Autodesk Fusion 360 part; units mm, degrees
(part 5 of 5)
  spline S1555 degree 3 poles (12.9782, 1.8894) (13.0053, 1.745) (13.1136, 1.5194) (13.2129, 1.4021) knots 0 0 0 0 1 1 1 1
  spline S1556 degree 3 poles (13.2129, 1.4021) (13.3122, 1.2667) (13.3844, 1.0411) (13.3844, 0.8335) knots 0 0 0 0 1 1 1 1
  spline S1557 degree 3 poles (13.3844, 0.8335) (13.3844, 0.6349) (13.4205, 0.4815) (13.4746, 0.4815) knots 0 0 0 0 1 1 1 1
  spline S1558 degree 3 poles (13.4746, 0.4815) (13.5288, 0.4815) (13.5649, 0.8245) (13.5649, 1.3389) knots 0 0 0 0 1 1 1 1
  spline S1559 degree 3 poles (13.2039, 0.7523) (13.2039, 0.8696) (13.1587, 0.9147) (13.0685, 0.8786) knots 0 0 0 0 1 1 1 1
  spline S1560 degree 3 poles (13.0685, 0.8786) (12.9602, 0.8335) (12.9512, 0.7884) (13.0324, 0.6981) knots 0 0 0 0 1 1 1 1
  spline S1561 degree 3 poles (13.0324, 0.6981) (13.1678, 0.5266) (13.2039, 0.5357) (13.2039, 0.7523) knots 0 0 0 0 1 1 1 1
  spline S1562 degree 3 poles (10.5866, 1.2577) (10.5234, 1.4021) (10.5234, 1.5465) (10.5866, 1.6548) knots 0 0 0 0 1 1 1 1
  spline S1563 degree 3 poles (10.5866, 1.6548) (10.7039, 1.8714) (10.7039, 2.1963) (10.5956, 2.1963) knots 0 0 0 0 1 1 1 1
  spline S1564 degree 3 poles (10.5956, 2.1963) (10.5505, 2.1963) (10.4783, 2.2775) (10.4512, 2.3858) knots 0 0 0 0 1 1 1 1
  spline S1565 degree 3 poles (10.4512, 2.3858) (10.3971, 2.5573) (10.3881, 2.5663) (10.2707, 2.4038) knots 0 0 0 0 1 1 1 1
  spline S1566 degree 3 poles (10.2707, 2.4038) (10.1895, 2.3046) (10.1805, 2.2053) (10.2346, 2.1602) knots 0 0 0 0 1 1 1 1
  spline S1567 degree 3 poles (10.2346, 2.1602) (10.2798, 2.106) (10.3159, 1.9345) (10.3159, 1.7721) knots 0 0 0 0 1 1 1 1
  spline S1568 degree 3 poles (10.3159, 1.7721) (10.3159, 1.4562) (10.4783, 1.023) (10.5956, 1.023) knots 0 0 0 0 1 1 1 1
  spline S1569 degree 3 poles (10.5956, 1.023) (10.6408, 1.023) (10.6317, 1.1313) (10.5866, 1.2577) knots 0 0 0 0 1 1 1 1
  spline S1570 degree 3 poles (12.8338, 1.5284) (12.8338, 1.6277) (12.8068, 1.6548) (12.7797, 1.5826) knots 0 0 0 0 1 1 1 1
  spline S1571 degree 3 poles (12.7797, 1.5826) (12.7526, 1.5194) (12.7616, 1.4382) (12.7887, 1.4111) knots 0 0 0 0 1 1 1 1
  spline S1572 degree 3 poles (12.7887, 1.4111) (12.8158, 1.375) (12.8429, 1.4291) (12.8338, 1.5284) knots 0 0 0 0 1 1 1 1
  spline S1573 degree 3 poles (11.3537, 2.9002) (11.3176, 3.0356) (11.3718, 3.0897) (11.5974, 3.1619) knots 0 0 0 0 1 1 1 1
  line L88 (11.5974, 3.1619) -> (11.8952, 3.2612)
  line L89 (11.8952, 3.2612) -> (11.5794, 3.2702)
  spline S1574 degree 3 poles (11.5794, 3.2702) (11.2003, 3.2793) (10.5595, 3.0717) (10.5144, 2.9183) knots 0 0 0 0 1 1 1 1
  spline S1575 degree 3 poles (10.5144, 2.9183) (10.4873, 2.837) (10.5686, 2.819) (10.8032, 2.8461) knots 0 0 0 0 1 1 1 1
  spline S1576 degree 3 poles (10.8032, 2.8461) (10.9837, 2.8641) (11.1281, 2.8461) (11.1281, 2.81) knots 0 0 0 0 1 1 1 1
  spline S1577 degree 3 poles (11.1281, 2.81) (11.1281, 2.7739) (11.1913, 2.7378) (11.2725, 2.7378) knots 0 0 0 0 1 1 1 1
  spline S1578 degree 3 poles (11.2725, 2.7378) (11.3628, 2.7378) (11.3898, 2.7919) (11.3537, 2.9002) knots 0 0 0 0 1 1 1 1
  spline S1579 degree 3 poles (10.1083, 3.0175) (10.1263, 3.198) (10.1173, 3.198) (9.9458, 3.0536) knots 0 0 0 0 1 1 1 1
  spline S1580 degree 3 poles (9.9458, 3.0536) (9.7292, 2.8551) (9.7292, 2.828) (9.9368, 2.828) knots 0 0 0 0 1 1 1 1
  spline S1581 degree 3 poles (9.9368, 2.828) (10.0361, 2.828) (10.0993, 2.9002) (10.1083, 3.0175) knots 0 0 0 0 1 1 1 1
  spline S1582 degree 3 poles (13.2941, 3.0446) (13.2941, 3.198) (13.0865, 3.2883) (12.9331, 3.189) knots 0 0 0 0 1 1 1 1
  spline S1583 degree 3 poles (12.9331, 3.189) (12.8429, 3.1349) (12.8609, 3.0897) (13.0053, 3.0175) knots 0 0 0 0 1 1 1 1
  spline S1584 degree 3 poles (13.0053, 3.0175) (13.249, 2.8912) (13.2941, 2.8912) (13.2941, 3.0446) knots 0 0 0 0 1 1 1 1
  spline S1585 degree 3 poles (-8.6727, -4.41) (-8.6366, -4.3017) (-8.5825, -4.2115) (-8.5374, -4.2115) knots 0 0 0 0 1 1 1 1
  spline S1586 degree 3 poles (-8.5374, -4.2115) (-8.4922, -4.2115) (-8.4561, -4.1483) (-8.4561, -4.0671) knots 0 0 0 0 1 1 1 1
  spline S1587 degree 3 poles (-8.4561, -4.0671) (-8.4561, -3.9498) (-8.5103, -3.9678) (-8.6998, -4.1573) knots 0 0 0 0 1 1 1 1
  spline S1588 degree 3 poles (-8.6998, -4.1573) (-8.8803, -4.3469) (-8.9164, -4.4191) (-8.8262, -4.5093) knots 0 0 0 0 1 1 1 1
  spline S1589 degree 3 poles (-8.8262, -4.5093) (-8.7449, -4.5905) (-8.7088, -4.5725) (-8.6727, -4.41) knots 0 0 0 0 1 1 1 1
  spline S1590 degree 3 poles (-9.864, -4.41) (-9.837, -4.3559) (-9.855, -4.2837) (-9.9092, -4.2566) knots 0 0 0 0 1 1 1 1
  spline S1591 degree 3 poles (-9.9092, -4.2566) (-10.0445, -4.1664) (-10.1348, -4.2837) (-10.0175, -4.401) knots 0 0 0 0 1 1 1 1
  spline S1592 degree 3 poles (-10.0175, -4.401) (-9.9543, -4.4642) (-9.9001, -4.4642) (-9.864, -4.41) knots 0 0 0 0 1 1 1 1
  spline S1593 degree 3 poles (-8.6637, -3.4895) (-8.6818, -3.3) (-8.7449, -3.2548) (-9.142, -3.1646) knots 0 0 0 0 1 1 1 1
  spline S1594 degree 3 poles (-9.142, -3.1646) (-9.6023, -3.0653) (-9.6113, -3.0653) (-9.6113, -3.2729) knots 0 0 0 0 1 1 1 1
  spline S1595 degree 3 poles (-9.6113, -3.2729) (-9.6113, -3.4263) (-9.5572, -3.4895) (-9.4399, -3.4895) knots 0 0 0 0 1 1 1 1
  spline S1596 degree 3 poles (-9.4399, -3.4895) (-9.3496, -3.4895) (-9.2594, -3.5256) (-9.2233, -3.5797) knots 0 0 0 0 1 1 1 1
  spline S1597 degree 3 poles (-9.2233, -3.5797) (-9.1962, -3.6339) (-9.0879, -3.6339) (-8.9525, -3.5797) knots 0 0 0 0 1 1 1 1
  spline S1598 degree 3 poles (-8.9525, -3.5797) (-8.8081, -3.5256) (-8.7269, -3.5346) (-8.6908, -3.6068) knots 0 0 0 0 1 1 1 1
  spline S1599 degree 3 poles (-8.6908, -3.6068) (-8.6637, -3.67) (-8.6547, -3.6158) (-8.6637, -3.4895) knots 0 0 0 0 1 1 1 1
  spline S1600 degree 3 poles (24.9363, -2.6321) (24.9363, -2.5058) (24.9724, -2.4065) (25.0266, -2.4065) knots 0 0 0 0 1 1 1 1
  spline S1601 degree 3 poles (25.0266, -2.4065) (25.0717, -2.4065) (25.1168, -2.3704) (25.1168, -2.3162) knots 0 0 0 0 1 1 1 1
  spline S1602 degree 3 poles (25.1168, -2.3162) (25.1168, -2.1809) (24.9724, -2.2079) (24.81, -2.3704) knots 0 0 0 0 1 1 1 1
  spline S1603 degree 3 poles (24.81, -2.3704) (24.6295, -2.5509) (24.6205, -2.8577) (24.801, -2.8577) knots 0 0 0 0 1 1 1 1
  spline S1604 degree 3 poles (24.801, -2.8577) (24.8822, -2.8577) (24.9363, -2.7765) (24.9363, -2.6321) knots 0 0 0 0 1 1 1 1
  spline S1605 degree 3 poles (-26.3798, -2.587) (-26.1542, -2.5509) (-26.1812, -2.5238) (-26.6415, -2.4245) knots 0 0 0 0 1 1 1 1
  spline S1606 degree 3 poles (-26.6415, -2.4245) (-27.165, -2.2982) (-27.4086, -2.3614) (-27.2733, -2.578) knots 0 0 0 0 1 1 1 1
  spline S1607 degree 3 poles (-27.2733, -2.578) (-27.2191, -2.6772) (-26.8852, -2.6863) (-26.3798, -2.587) knots 0 0 0 0 1 1 1 1
  spline S1608 degree 3 poles (-24.1596, -2.4877) (-24.1596, -2.4155) (-24.4936, -2.3162) (-24.7282, -2.3162) knots 0 0 0 0 1 1 1 1
  spline S1609 degree 3 poles (-24.7282, -2.3162) (-24.8726, -2.3162) (-24.8726, -2.3343) (-24.7643, -2.4426) knots 0 0 0 0 1 1 1 1
  spline S1610 degree 3 poles (-24.7643, -2.4426) (-24.647, -2.5689) (-24.1596, -2.596) (-24.1596, -2.4877) knots 0 0 0 0 1 1 1 1
  spline S1611 degree 3 poles (-23.7084, -2.4065) (-23.7084, -2.3614) (-23.7535, -2.3162) (-23.7986, -2.3162) knots 0 0 0 0 1 1 1 1
  spline S1612 degree 3 poles (-23.7986, -2.3162) (-23.8528, -2.3162) (-23.8889, -2.3614) (-23.8889, -2.4065) knots 0 0 0 0 1 1 1 1
  spline S1613 degree 3 poles (-23.8889, -2.4065) (-23.8889, -2.4606) (-23.8528, -2.4967) (-23.7986, -2.4967) knots 0 0 0 0 1 1 1 1
  spline S1614 degree 3 poles (-23.7986, -2.4967) (-23.7535, -2.4967) (-23.7084, -2.4606) (-23.7084, -2.4065) knots 0 0 0 0 1 1 1 1
  spline S1615 degree 3 poles (-25.6758, -1.2242) (-25.5224, -1.0618) (-25.5224, -1.0527) (-25.6849, -1.0527) knots 0 0 0 0 1 1 1 1
  spline S1616 degree 3 poles (-25.6849, -1.0527) (-25.8924, -1.0527) (-26.5152, -1.3145) (-26.3256, -1.3235) knots 0 0 0 0 1 1 1 1
  spline S1617 degree 3 poles (-26.3256, -1.3235) (-26.2534, -1.3235) (-26.109, -1.3415) (-26.0098, -1.3686) knots 0 0 0 0 1 1 1 1
  spline S1618 degree 3 poles (-26.0098, -1.3686) (-25.9015, -1.3867) (-25.7661, -1.3325) (-25.6758, -1.2242) knots 0 0 0 0 1 1 1 1
  spline S1619 degree 3 poles (-26.3617, -0.8) (-26.3888, -0.7549) (-26.5693, -0.6917) (-26.7679, -0.6556) knots 0 0 0 0 1 1 1 1
  spline S1620 degree 3 poles (-26.7679, -0.6556) (-26.9664, -0.6286) (-27.1379, -0.5564) (-27.1559, -0.5022) knots 0 0 0 0 1 1 1 1
  spline S1621 degree 3 poles (-27.1559, -0.5022) (-27.2011, -0.3578) (-27.5079, -0.5203) (-27.4808, -0.6827) knots 0 0 0 0 1 1 1 1
  spline S1622 degree 3 poles (-27.4808, -0.6827) (-27.4628, -0.791) (-27.3184, -0.8361) (-26.8852, -0.8542) knots 0 0 0 0 1 1 1 1
  spline S1623 degree 3 poles (-26.8852, -0.8542) (-26.5513, -0.8722) (-26.3347, -0.8452) (-26.3617, -0.8) knots 0 0 0 0 1 1 1 1
  spline S1624 degree 3 poles (-23.9791, -0.6827) (-23.9791, -0.6376) (-24.0243, -0.6195) (-24.0694, -0.6466) knots 0 0 0 0 1 1 1 1
  spline S1625 degree 3 poles (-24.0694, -0.6466) (-24.1235, -0.6737) (-24.1596, -0.7188) (-24.1596, -0.7459) knots 0 0 0 0 1 1 1 1
  spline S1626 degree 3 poles (-24.1596, -0.7459) (-24.1596, -0.7639) (-24.1235, -0.782) (-24.0694, -0.782) knots 0 0 0 0 1 1 1 1
  spline S1627 degree 3 poles (-24.0694, -0.782) (-24.0243, -0.782) (-23.9791, -0.7369) (-23.9791, -0.6827) knots 0 0 0 0 1 1 1 1
  spline S1628 degree 3 poles (-25.2426, -0.6015) (-25.2426, -0.5564) (-25.2878, -0.5112) (-25.3329, -0.5112) knots 0 0 0 0 1 1 1 1
  spline S1629 degree 3 poles (-25.3329, -0.5112) (-25.387, -0.5112) (-25.4231, -0.5564) (-25.4231, -0.6015) knots 0 0 0 0 1 1 1 1
  spline S1630 degree 3 poles (-25.4231, -0.6015) (-25.4231, -0.6556) (-25.387, -0.6917) (-25.3329, -0.6917) knots 0 0 0 0 1 1 1 1
  spline S1631 degree 3 poles (-25.3329, -0.6917) (-25.2878, -0.6917) (-25.2426, -0.6556) (-25.2426, -0.6015) knots 0 0 0 0 1 1 1 1
  spline S1632 degree 3 poles (-23.3474, -0.4661) (-23.2571, -0.3668) (-23.2571, -0.2946) (-23.3293, -0.2224) knots 0 0 0 0 1 1 1 1
  spline S1633 degree 3 poles (-23.3293, -0.2224) (-23.4647, -0.0871) (-23.7264, -0.2044) (-23.6903, -0.3939) knots 0 0 0 0 1 1 1 1
  spline S1634 degree 3 poles (-23.6903, -0.3939) (-23.6542, -0.6015) (-23.4918, -0.6376) (-23.3474, -0.4661) knots 0 0 0 0 1 1 1 1
  spline S1635 degree 3 poles (-24.7643, -0.4481) (-24.665, -0.3578) (-24.8907, -0.1502) (-25.0982, -0.1502) knots 0 0 0 0 1 1 1 1
  spline S1636 degree 3 poles (-25.0982, -0.1502) (-25.1975, -0.1502) (-25.3509, -0.1863) (-25.4231, -0.2405) knots 0 0 0 0 1 1 1 1
  spline S1637 degree 3 poles (-25.4231, -0.2405) (-25.5405, -0.3127) (-25.5405, -0.3217) (-25.4231, -0.3668) knots 0 0 0 0 1 1 1 1
  spline S1638 degree 3 poles (-25.4231, -0.3668) (-25.0982, -0.4661) (-24.8094, -0.5022) (-24.7643, -0.4481) knots 0 0 0 0 1 1 1 1
  spline S1639 degree 3 poles (-22.5803, -0.2405) (-22.5532, -0.1954) (-22.5622, -0.1502) (-22.6164, -0.1502) knots 0 0 0 0 1 1 1 1
  spline S1640 degree 3 poles (-22.6164, -0.1502) (-22.6615, -0.1502) (-22.7337, -0.1954) (-22.7608, -0.2405) knots 0 0 0 0 1 1 1 1
  spline S1641 degree 3 poles (-22.7608, -0.2405) (-22.7878, -0.2946) (-22.7788, -0.3307) (-22.7247, -0.3307) knots 0 0 0 0 1 1 1 1
  spline S1642 degree 3 poles (-22.7247, -0.3307) (-22.6795, -0.3307) (-22.6073, -0.2946) (-22.5803, -0.2405) knots 0 0 0 0 1 1 1 1
  spline S1643 degree 3 poles (-23.7986, -0.2495) (-23.7986, -0.1502) (-24.0333, -0.051) (-24.1055, -0.1232) knots 0 0 0 0 1 1 1 1
  spline S1644 degree 3 poles (-24.1055, -0.1232) (-24.2138, -0.2315) (-24.1506, -0.3307) (-23.9791, -0.3307) knots 0 0 0 0 1 1 1 1
  spline S1645 degree 3 poles (-23.9791, -0.3307) (-23.8799, -0.3307) (-23.7986, -0.2946) (-23.7986, -0.2495) knots 0 0 0 0 1 1 1 1
  spline S1646 degree 3 poles (-24.4123, -0.0871) (-24.4755, -0.06) (-24.5567, -0.069) (-24.5838, -0.0961) knots 0 0 0 0 1 1 1 1
  spline S1647 degree 3 poles (-24.5838, -0.0961) (-24.6199, -0.1232) (-24.5658, -0.1502) (-24.4665, -0.1412) knots 0 0 0 0 1 1 1 1
  spline S1648 degree 3 poles (-24.4665, -0.1412) (-24.3672, -0.1412) (-24.3401, -0.1141) (-24.4123, -0.0871) knots 0 0 0 0 1 1 1 1
  spline S1649 degree 3 poles (-26.804, 0.0032) (-26.8852, 0.0844) (-26.9754, 0.1295) (-27.0115, 0.1025) knots 0 0 0 0 1 1 1 1
  spline S1650 degree 3 poles (-27.0115, 0.1025) (-27.1018, 0.0122) (-26.9574, -0.1502) (-26.7949, -0.1502) knots 0 0 0 0 1 1 1 1
  spline S1651 degree 3 poles (-26.7949, -0.1502) (-26.6596, -0.1502) (-26.6596, -0.1412) (-26.804, 0.0032) knots 0 0 0 0 1 1 1 1
  spline S1652 degree 3 poles (-21.6868, 0.5627) (-21.5695, 0.6981) (-21.5604, 0.7432) (-21.6507, 0.7703) knots 0 0 0 0 1 1 1 1
  spline S1653 degree 3 poles (-21.6507, 0.7703) (-21.7409, 0.8064) (-21.7409, 0.8515) (-21.6326, 0.9869) knots 0 0 0 0 1 1 1 1
  spline S1654 degree 3 poles (-21.6326, 0.9869) (-21.5063, 1.1494) (-21.5063, 1.1494) (-21.7229, 1.014) knots 0 0 0 0 1 1 1 1
  spline S1655 degree 3 poles (-21.7229, 1.014) (-21.8673, 0.9147) (-21.9485, 0.7793) (-21.9485, 0.6259) knots 0 0 0 0 1 1 1 1
  spline S1656 degree 3 poles (-21.9485, 0.6259) (-21.9575, 0.3461) (-21.8944, 0.3281) (-21.6868, 0.5627) knots 0 0 0 0 1 1 1 1
  spline S1657 degree 3 poles (-22.1741, 1.1584) (-22.0839, 1.2667) (-22.0839, 1.2938) (-22.2012, 1.2938) knots 0 0 0 0 1 1 1 1
  spline S1658 degree 3 poles (-22.2012, 1.2938) (-22.3727, 1.2938) (-22.481, 1.1494) (-22.3637, 1.0772) knots 0 0 0 0 1 1 1 1
  spline S1659 degree 3 poles (-22.3637, 1.0772) (-22.3185, 1.0501) (-22.2373, 1.0862) (-22.1741, 1.1584) knots 0 0 0 0 1 1 1 1
  spline S1660 degree 3 poles (-19.8998, 2.088) (-19.6742, 2.2685) (-19.4396, 2.5121) (-19.3944, 2.6114) knots 0 0 0 0 1 1 1 1
  spline S1661 degree 3 poles (-19.3944, 2.6114) (-19.3042, 2.7919) (-19.3313, 2.81) (-19.7645, 2.8551) knots 0 0 0 0 1 1 1 1
  spline S1662 degree 3 poles (-19.7645, 2.8551) (-20.2789, 2.9183) (-20.4052, 2.8731) (-20.1706, 2.7017) knots 0 0 0 0 1 1 1 1
  spline S1663 degree 3 poles (-20.1706, 2.7017) (-19.972, 2.5573) (-20.0533, 2.467) (-20.3601, 2.467) knots 0 0 0 0 1 1 1 1
  line L90 (-20.3601, 2.467) -> (-20.5857, 2.467)
  line L91 (-20.5857, 2.467) -> (-20.3782, 2.3226)
  spline S1664 degree 3 poles (-20.3782, 2.3226) (-20.2157, 2.2053) (-20.1525, 2.1963) (-20.0984, 2.2865) knots 0 0 0 0 1 1 1 1
  spline S1665 degree 3 poles (-20.0984, 2.2865) (-20.0623, 2.3497) (-20.0081, 2.3587) (-19.9811, 2.3136) knots 0 0 0 0 1 1 1 1
  spline S1666 degree 3 poles (-19.9811, 2.3136) (-19.945, 2.2594) (-20.0262, 2.1782) (-20.1435, 2.1241) knots 0 0 0 0 1 1 1 1
  spline S1667 degree 3 poles (-20.1435, 2.1241) (-20.2699, 2.0609) (-20.3691, 1.9616) (-20.3691, 1.8804) knots 0 0 0 0 1 1 1 1
  spline S1668 degree 3 poles (-20.3691, 1.8804) (-20.3691, 1.7089) (-20.3962, 1.6999) (-19.8998, 2.088) knots 0 0 0 0 1 1 1 1
  spline S1669 degree 3 poles (-18.6995, 2.6475) (-18.2573, 2.8551) (-17.9685, 3.0807) (-18.0407, 3.1529) knots 0 0 0 0 1 1 1 1
  spline S1670 degree 3 poles (-18.0407, 3.1529) (-18.0768, 3.18) (-18.1761, 3.1619) (-18.2753, 3.1078) knots 0 0 0 0 1 1 1 1
  spline S1671 degree 3 poles (-18.2753, 3.1078) (-18.4829, 2.9995) (-18.7446, 3.0627) (-18.7446, 3.2251) knots 0 0 0 0 1 1 1 1
  spline S1672 degree 3 poles (-18.7446, 3.2251) (-18.7446, 3.2883) (-18.8981, 3.3244) (-19.1417, 3.3244) knots 0 0 0 0 1 1 1 1
  spline S1673 degree 3 poles (-19.1417, 3.3244) (-19.584, 3.3244) (-19.7554, 3.2341) (-19.4847, 3.1529) knots 0 0 0 0 1 1 1 1
  spline S1674 degree 3 poles (-19.4847, 3.1529) (-19.3854, 3.1168) (-19.2771, 3.0356) (-19.25, 2.9634) knots 0 0 0 0 1 1 1 1
  spline S1675 degree 3 poles (-19.25, 2.9634) (-19.223, 2.8912) (-19.1417, 2.828) (-19.0605, 2.828) knots 0 0 0 0 1 1 1 1
  spline S1676 degree 3 poles (-19.0605, 2.828) (-18.88, 2.828) (-18.889, 2.6746) (-19.0876, 2.5663) knots 0 0 0 0 1 1 1 1
  spline S1677 degree 3 poles (-19.0876, 2.5663) (-19.3583, 2.4038) (-19.0786, 2.467) (-18.6995, 2.6475) knots 0 0 0 0 1 1 1 1
  spline S1678 degree 3 poles (-20.9106, 2.9273) (-20.9106, 2.9724) (-20.9558, 2.9905) (-21.0009, 2.9634) knots 0 0 0 0 1 1 1 1
  spline S1679 degree 3 poles (-21.0009, 2.9634) (-21.055, 2.9363) (-21.0911, 2.8912) (-21.0911, 2.8641) knots 0 0 0 0 1 1 1 1
  spline S1680 degree 3 poles (-21.0911, 2.8641) (-21.0911, 2.8461) (-21.055, 2.828) (-21.0009, 2.828) knots 0 0 0 0 1 1 1 1
  spline S1681 degree 3 poles (-21.0009, 2.828) (-20.9558, 2.828) (-20.9106, 2.8731) (-20.9106, 2.9273) knots 0 0 0 0 1 1 1 1
  spline S1682 degree 3 poles (-17.1743, 3.3154) (-17.0299, 3.3785) (-16.9577, 3.4598) (-17.0118, 3.4959) knots 0 0 0 0 1 1 1 1
  spline S1683 degree 3 poles (-17.0118, 3.4959) (-17.1201, 3.559) (-17.5263, 3.4237) (-17.6165, 3.2883) knots 0 0 0 0 1 1 1 1
  spline S1684 degree 3 poles (-17.6165, 3.2883) (-17.6887, 3.1619) (-17.4992, 3.171) (-17.1743, 3.3154) knots 0 0 0 0 1 1 1 1
  spline S1685 degree 3 poles (19.9004, -0.8361) (20.0177, -0.7459) (20.0358, -0.7008) (19.9546, -0.6195) knots 0 0 0 0 1 1 1 1
  spline S1686 degree 3 poles (19.9546, -0.6195) (19.8914, -0.5564) (19.8011, -0.5112) (19.747, -0.5112) knots 0 0 0 0 1 1 1 1
  spline S1687 degree 3 poles (19.747, -0.5112) (19.6567, -0.5112) (19.3409, -0.8271) (19.3409, -0.9174) knots 0 0 0 0 1 1 1 1
  spline S1688 degree 3 poles (19.3409, -0.9174) (19.3409, -1.0076) (19.756, -0.9535) (19.9004, -0.8361) knots 0 0 0 0 1 1 1 1
  spline S1689 degree 3 poles (18.3481, -0.8722) (18.3481, -0.8271) (18.303, -0.782) (18.2488, -0.782) knots 0 0 0 0 1 1 1 1
  spline S1690 degree 3 poles (18.2488, -0.782) (18.2037, -0.782) (18.1857, -0.8271) (18.2127, -0.8722) knots 0 0 0 0 1 1 1 1
  spline S1691 degree 3 poles (18.2127, -0.8722) (18.2398, -0.9264) (18.2849, -0.9625) (18.312, -0.9625) knots 0 0 0 0 1 1 1 1
  spline S1692 degree 3 poles (18.312, -0.9625) (18.3301, -0.9625) (18.3481, -0.9264) (18.3481, -0.8722) knots 0 0 0 0 1 1 1 1
  spline S1693 degree 3 poles (19.2957, -0.6917) (19.3679, -0.5744) (19.1062, -0.4751) (18.9618, -0.5654) knots 0 0 0 0 1 1 1 1
  spline S1694 degree 3 poles (18.9618, -0.5654) (18.8986, -0.6105) (18.7723, -0.6286) (18.673, -0.6105) knots 0 0 0 0 1 1 1 1
  spline S1695 degree 3 poles (18.673, -0.6105) (18.5737, -0.6015) (18.5286, -0.6286) (18.5647, -0.6827) knots 0 0 0 0 1 1 1 1
  spline S1696 degree 3 poles (18.5647, -0.6827) (18.6459, -0.8091) (19.2235, -0.8091) (19.2957, -0.6917) knots 0 0 0 0 1 1 1 1
  spline S1697 degree 3 poles (17.6712, -0.421) (17.6442, -0.3759) (17.5539, -0.3307) (17.4817, -0.3307) knots 0 0 0 0 1 1 1 1
  spline S1698 degree 3 poles (17.4817, -0.3307) (17.4095, -0.3307) (17.3554, -0.3759) (17.3554, -0.421) knots 0 0 0 0 1 1 1 1
  spline S1699 degree 3 poles (17.3554, -0.421) (17.3554, -0.4751) (17.4366, -0.5112) (17.5449, -0.5112) knots 0 0 0 0 1 1 1 1
  spline S1700 degree 3 poles (17.5449, -0.5112) (17.6442, -0.5112) (17.6983, -0.4751) (17.6712, -0.421) knots 0 0 0 0 1 1 1 1
  spline S1701 degree 3 poles (22.996, 1.4743) (23.023, 1.5194) (23.014, 1.5645) (22.9599, 1.5645) knots 0 0 0 0 1 1 1 1
  spline S1702 degree 3 poles (22.9599, 1.5645) (22.9147, 1.5645) (22.8425, 1.5194) (22.8155, 1.4743) knots 0 0 0 0 1 1 1 1
  spline S1703 degree 3 poles (22.8155, 1.4743) (22.7884, 1.4201) (22.7974, 1.384) (22.8516, 1.384) knots 0 0 0 0 1 1 1 1
  spline S1704 degree 3 poles (22.8516, 1.384) (22.8967, 1.384) (22.9689, 1.4201) (22.996, 1.4743) knots 0 0 0 0 1 1 1 1
  spline S1705 degree 3 poles (22.8877, 1.754) (23.014, 1.8262) (23.0321, 1.8804) (22.9418, 1.9797) knots 0 0 0 0 1 1 1 1
  spline S1706 degree 3 poles (22.9418, 1.9797) (22.8064, 2.1511) (22.5357, 2.1421) (22.4635, 1.9616) knots 0 0 0 0 1 1 1 1
  spline S1707 degree 3 poles (22.4635, 1.9616) (22.3552, 1.6818) (22.5718, 1.5735) (22.8877, 1.754) knots 0 0 0 0 1 1 1 1
  spline S1708 degree 3 poles (23.0411, 2.1963) (23.0411, 2.2414) (22.996, 2.2865) (22.9508, 2.2865) knots 0 0 0 0 1 1 1 1
  spline S1709 degree 3 poles (22.9508, 2.2865) (22.8967, 2.2865) (22.8606, 2.2414) (22.8606, 2.1963) knots 0 0 0 0 1 1 1 1
  spline S1710 degree 3 poles (22.8606, 2.1963) (22.8606, 2.1421) (22.8967, 2.106) (22.9508, 2.106) knots 0 0 0 0 1 1 1 1
  spline S1711 degree 3 poles (22.9508, 2.106) (22.996, 2.106) (23.0411, 2.1421) (23.0411, 2.1963) knots 0 0 0 0 1 1 1 1
  spline S1712 degree 3 poles (25.2973, 2.9092) (25.2973, 3.0266) (25.1078, 3.0807) (24.9093, 3.0266) knots 0 0 0 0 1 1 1 1
  spline S1713 degree 3 poles (24.9093, 3.0266) (24.7739, 2.9905) (24.7649, 2.9634) (24.8641, 2.9092) knots 0 0 0 0 1 1 1 1
  spline S1714 degree 3 poles (24.8641, 2.9092) (25.0176, 2.8009) (25.2973, 2.81) (25.2973, 2.9092) knots 0 0 0 0 1 1 1 1
  spline S1715 degree 3 poles (-28.8526, 0.1656) (-28.8526, 0.2378) (-28.9158, 0.301) (-28.988, 0.301) knots 0 0 0 0 1 1 1 1
  spline S1716 degree 3 poles (-28.988, 0.301) (-29.0602, 0.301) (-29.1234, 0.2378) (-29.1234, 0.1656) knots 0 0 0 0 1 1 1 1
  spline S1717 degree 3 poles (-29.1234, 0.1656) (-29.1234, 0.0934) (-29.0602, 0.0303) (-28.988, 0.0303) knots 0 0 0 0 1 1 1 1
  spline S1718 degree 3 poles (-28.988, 0.0303) (-28.9158, 0.0303) (-28.8526, 0.0934) (-28.8526, 0.1656) knots 0 0 0 0 1 1 1 1
  spline S1719 degree 3 poles (-28.7895, 0.9689) (-28.8165, 1.3118) (-29.349, 1.7631) (-29.6468, 1.6909) knots 0 0 0 0 1 1 1 1
  spline S1720 degree 3 poles (-29.6468, 1.6909) (-29.8815, 1.6277) (-29.9086, 1.5194) (-29.692, 1.4382) knots 0 0 0 0 1 1 1 1
  spline S1721 degree 3 poles (-29.692, 1.4382) (-29.3219, 1.3028) (-28.8978, 1.014) (-28.8346, 0.8696) knots 0 0 0 0 1 1 1 1
  spline S1722 degree 3 poles (-28.8346, 0.8696) (-28.7895, 0.7523) (-28.7714, 0.7884) (-28.7895, 0.9689) knots 0 0 0 0 1 1 1 1
  spline S1723 degree 3 poles (23.4292, 3.8659) (23.6097, 4.0915) (23.6458, 4.1818) (23.5465, 4.1818) knots 0 0 0 0 1 1 1 1
  spline S1724 degree 3 poles (23.5465, 4.1818) (23.357, 4.1818) (23.1313, 3.9291) (23.1313, 3.7215) knots 0 0 0 0 1 1 1 1
  spline S1725 degree 3 poles (23.1313, 3.7215) (23.1313, 3.6312) (23.1404, 3.55) (23.1494, 3.55) knots 0 0 0 0 1 1 1 1
  spline S1726 degree 3 poles (23.1494, 3.55) (23.1674, 3.55) (23.2938, 3.6944) (23.4292, 3.8659) knots 0 0 0 0 1 1 1 1
  spline S1727 degree 3 poles (26.5247, 3.8659) (26.3081, 4.0283) (26.0825, 4.0464) (26.1276, 3.8839) knots 0 0 0 0 1 1 1 1
  spline S1728 degree 3 poles (26.1276, 3.8839) (26.1547, 3.8298) (26.2901, 3.7666) (26.4345, 3.7486) knots 0 0 0 0 1 1 1 1
  spline S1729 degree 3 poles (26.4345, 3.7486) (26.6872, 3.7305) (26.6872, 3.7305) (26.5247, 3.8659) knots 0 0 0 0 1 1 1 1
  spline S1730 degree 3 poles (25.8749, 4.0464) (25.8388, 4.1186) (25.7847, 4.1818) (25.7486, 4.1818) knots 0 0 0 0 1 1 1 1
  spline S1731 degree 3 poles (25.7486, 4.1818) (25.7125, 4.1818) (25.6583, 4.1186) (25.6222, 4.0464) knots 0 0 0 0 1 1 1 1
  spline S1732 degree 3 poles (25.6222, 4.0464) (25.5861, 3.9561) (25.6313, 3.911) (25.7486, 3.911) knots 0 0 0 0 1 1 1 1
  spline S1733 degree 3 poles (25.7486, 3.911) (25.8659, 3.911) (25.911, 3.9561) (25.8749, 4.0464) knots 0 0 0 0 1 1 1 1
  spline S1734 degree 3 poles (26.2901, 4.2991) (26.2901, 4.3803) (26.3442, 4.4615) (26.3984, 4.4886) knots 0 0 0 0 1 1 1 1
  spline S1735 degree 3 poles (26.3984, 4.4886) (26.4616, 4.5157) (26.3894, 4.5247) (26.245, 4.5157) knots 0 0 0 0 1 1 1 1
  spline S1736 degree 3 poles (26.245, 4.5157) (25.9471, 4.4976) (25.8659, 4.254) (26.1276, 4.1998) knots 0 0 0 0 1 1 1 1
  spline S1737 degree 3 poles (26.1276, 4.1998) (26.2269, 4.1818) (26.2901, 4.2269) (26.2901, 4.2991) knots 0 0 0 0 1 1 1 1
  spline S1738 degree 3 poles (21.1819, -7.6861) (21.209, -7.6049) (21.2361, -6.9641) (21.2361, -6.2782) knots 0 0 0 0 1 1 1 1
  spline S1739 degree 3 poles (21.2361, -6.2782) (21.2361, -5.0689) (21.2271, -5.0147) (21.0646, -5.0689) knots 0 0 0 0 1 1 1 1
  spline S1740 degree 3 poles (21.0646, -5.0689) (20.9383, -5.105) (20.8751, -5.0689) (20.848, -4.9606) knots 0 0 0 0 1 1 1 1
  spline S1741 degree 3 poles (20.848, -4.9606) (20.8119, -4.8071) (20.8029, -4.8071) (20.7939, -4.9606) knots 0 0 0 0 1 1 1 1
  spline S1742 degree 3 poles (20.7939, -4.9606) (20.7758, -5.2223) (20.5141, -5.1411) (20.5051, -4.8703) knots 0 0 0 0 1 1 1 1
  spline S1743 degree 3 poles (20.5051, -4.8703) (20.4961, -4.6898) (20.469, -4.7259) (20.4148, -5.0147) knots 0 0 0 0 1 1 1 1
  spline S1744 degree 3 poles (20.4148, -5.0147) (20.3246, -5.484) (20.3607, -5.5652) (20.6585, -5.5652) knots 0 0 0 0 1 1 1 1
  spline S1745 degree 3 poles (20.6585, -5.5652) (20.8209, -5.5652) (20.8751, -5.6104) (20.8751, -5.7728) knots 0 0 0 0 1 1 1 1
  spline S1746 degree 3 poles (20.8751, -5.7728) (20.8751, -6.0345) (20.7848, -6.1338) (20.6585, -6.0255) knots 0 0 0 0 1 1 1 1
  spline S1747 degree 3 poles (20.6585, -6.0255) (20.5321, -5.9172) (20.1982, -6.1428) (20.2885, -6.2782) knots 0 0 0 0 1 1 1 1
  spline S1748 degree 3 poles (20.2885, -6.2782) (20.3156, -6.3324) (20.4419, -6.3775) (20.5682, -6.3775) knots 0 0 0 0 1 1 1 1
  spline S1749 degree 3 poles (20.5682, -6.3775) (20.7758, -6.3775) (20.7848, -6.4046) (20.7848, -6.8739) knots 0 0 0 0 1 1 1 1
  spline S1750 degree 3 poles (20.7848, -6.8739) (20.7848, -7.4244) (20.5953, -7.5688) (20.4419, -7.1266) knots 0 0 0 0 1 1 1 1
  line L92 (20.4419, -7.1266) -> (20.3607, -6.8739)
  line L93 (20.3607, -6.8739) -> (20.2885, -7.2168)
  spline S1751 degree 3 poles (20.2885, -7.2168) (20.2073, -7.632) (20.2795, -7.7312) (20.7578, -7.7944) knots 0 0 0 0 1 1 1 1
  spline S1752 degree 3 poles (20.7578, -7.7944) (21.0466, -7.8305) (21.1278, -7.8125) (21.1819, -7.6861) knots 0 0 0 0 1 1 1 1
  spline S1753 degree 3 poles (25.9742, -7.641) (26.4796, -7.4424) (26.5338, -6.9009) (26.1547, -5.827) knots 0 0 0 0 1 1 1 1
  spline S1754 degree 3 poles (26.1547, -5.827) (26.0284, -5.4479) (25.9291, -4.9696) (25.9291, -4.6988) knots 0 0 0 0 1 1 1 1
  spline S1755 degree 3 poles (25.9291, -4.6988) (25.9291, -4.4371) (25.884, -4.1934) (25.8388, -4.1664) knots 0 0 0 0 1 1 1 1
  spline S1756 degree 3 poles (25.8388, -4.1664) (25.7847, -4.1303) (25.7486, -4.2386) (25.7486, -4.4371) knots 0 0 0 0 1 1 1 1
  spline S1757 degree 3 poles (25.7486, -4.4371) (25.7486, -4.6357) (25.7125, -4.744) (25.6583, -4.7079) knots 0 0 0 0 1 1 1 1
  spline S1758 degree 3 poles (25.6583, -4.7079) (25.6042, -4.6718) (25.5681, -4.7981) (25.5681, -5.0147) knots 0 0 0 0 1 1 1 1
  spline S1759 degree 3 poles (25.5681, -5.0147) (25.5681, -5.2133) (25.6042, -5.4028) (25.6583, -5.4299) knots 0 0 0 0 1 1 1 1
  spline S1760 degree 3 poles (25.6583, -5.4299) (25.7666, -5.5021) (25.7757, -5.9894) (25.6674, -6.0526) knots 0 0 0 0 1 1 1 1
  spline S1761 degree 3 poles (25.6674, -6.0526) (25.6222, -6.0887) (25.532, -6.0887) (25.4598, -6.0616) knots 0 0 0 0 1 1 1 1
  spline S1762 degree 3 poles (25.4598, -6.0616) (25.3154, -6.0075) (24.8461, -5.1862) (24.8461, -4.9876) knots 0 0 0 0 1 1 1 1
  spline S1763 degree 3 poles (24.8461, -4.9876) (24.8461, -4.9064) (24.801, -4.8432) (24.7558, -4.8432) knots 0 0 0 0 1 1 1 1
  spline S1764 degree 3 poles (24.7558, -4.8432) (24.7017, -4.8432) (24.6656, -4.744) (24.6656, -4.6176) knots 0 0 0 0 1 1 1 1
  spline S1765 degree 3 poles (24.6656, -4.6176) (24.6656, -4.4913) (24.6205, -4.392) (24.5753, -4.392) knots 0 0 0 0 1 1 1 1
  spline S1766 degree 3 poles (24.5753, -4.392) (24.467, -4.392) (24.467, -4.3739) (24.5663, -4.7349) knots 0 0 0 0 1 1 1 1
  spline S1767 degree 3 poles (24.5663, -4.7349) (24.6205, -4.8974) (24.6205, -5.123) (24.5844, -5.2313) knots 0 0 0 0 1 1 1 1
  spline S1768 degree 3 poles (24.5844, -5.2313) (24.5302, -5.3847) (24.5844, -5.5291) (24.8551, -5.8992) knots 0 0 0 0 1 1 1 1
  spline S1769 degree 3 poles (24.8551, -5.8992) (25.2432, -6.4136) (25.2793, -6.5399) (25.0717, -6.6121) knots 0 0 0 0 1 1 1 1
  spline S1770 degree 3 poles (25.0717, -6.6121) (24.9002, -6.6843) (24.9002, -7.0092) (25.0807, -7.2619) knots 0 0 0 0 1 1 1 1
  spline S1771 degree 3 poles (25.0807, -7.2619) (25.189, -7.4244) (25.6674, -7.7493) (25.7666, -7.7222) knots 0 0 0 0 1 1 1 1
  spline S1772 degree 3 poles (25.7666, -7.7222) (25.7847, -7.7222) (25.8749, -7.6861) (25.9742, -7.641) knots 0 0 0 0 1 1 1 1
  spline S1773 degree 3 poles (25.4959, -7.2258) (25.3876, -7.1536) (25.2973, -7.0363) (25.2973, -6.9822) knots 0 0 0 0 1 1 1 1
  spline S1774 degree 3 poles (25.2973, -6.9822) (25.2973, -6.8197) (25.7486, -6.3594) (25.8659, -6.4046) knots 0 0 0 0 1 1 1 1
  spline S1775 degree 3 poles (25.8659, -6.4046) (26.0374, -6.4587) (26.1006, -7.0905) (25.9562, -7.2439) knots 0 0 0 0 1 1 1 1
  spline S1776 degree 3 poles (25.9562, -7.2439) (25.7937, -7.4063) (25.7486, -7.4063) (25.4959, -7.2258) knots 0 0 0 0 1 1 1 1
  spline S1777 degree 3 poles (24.1782, -7.5417) (24.3226, -7.3793) (24.3497, -7.2258) (24.3317, -6.6031) knots 0 0 0 0 1 1 1 1
  spline S1778 degree 3 poles (24.3317, -6.6031) (24.3226, -6.1699) (24.2595, -5.7187) (24.1782, -5.5201) knots 0 0 0 0 1 1 1 1
  spline S1779 degree 3 poles (24.1782, -5.5201) (24.097, -5.3306) (24.0338, -5.0959) (24.0248, -4.9876) knots 0 0 0 0 1 1 1 1
  spline S1780 degree 3 poles (24.0248, -4.9876) (24.0248, -4.7981) (24.0248, -4.7981) (23.9436, -5.0057) knots 0 0 0 0 1 1 1 1
  spline S1781 degree 3 poles (23.9436, -5.0057) (23.8263, -5.2945) (23.6728, -5.2494) (23.6728, -4.9335) knots 0 0 0 0 1 1 1 1
  spline S1782 degree 3 poles (23.6728, -4.9335) (23.6728, -4.7891) (23.6277, -4.6627) (23.5826, -4.6627) knots 0 0 0 0 1 1 1 1
  spline S1783 degree 3 poles (23.5826, -4.6627) (23.5284, -4.6627) (23.4923, -4.7801) (23.4923, -4.9154) knots 0 0 0 0 1 1 1 1
  spline S1784 degree 3 poles (23.4923, -4.9154) (23.4923, -5.0508) (23.4472, -5.2133) (23.384, -5.2764) knots 0 0 0 0 1 1 1 1
  spline S1785 degree 3 poles (23.384, -5.2764) (23.3299, -5.3306) (23.2667, -5.7818) (23.2396, -6.3143) knots 0 0 0 0 1 1 1 1
  line L94 (23.2396, -6.3143) -> (23.2035, -7.2439)
  line L95 (23.2035, -7.2439) -> (23.4923, -7.4876)
  spline S1786 degree 3 poles (23.4923, -7.4876) (23.8353, -7.7854) (23.9526, -7.7944) (24.1782, -7.5417) knots 0 0 0 0 1 1 1 1
  spline S1787 degree 3 poles (23.6006, -7.0002) (23.5284, -6.8648) (23.5014, -6.5941) (23.5284, -6.2511) knots 0 0 0 0 1 1 1 1
  spline S1788 degree 3 poles (23.5284, -6.2511) (23.5826, -5.6645) (23.6097, -5.6104) (23.7902, -5.6826) knots 0 0 0 0 1 1 1 1
  spline S1789 degree 3 poles (23.7902, -5.6826) (23.9255, -5.7367) (24.0699, -6.9009) (23.9707, -7.1536) knots 0 0 0 0 1 1 1 1
  spline S1790 degree 3 poles (23.9707, -7.1536) (23.9075, -7.3341) (23.745, -7.271) (23.6006, -7.0002) knots 0 0 0 0 1 1 1 1
extrude "Extrude3" add sketch "Sketch3" along normal blind 2 contours A0 | S16 S17 S18 | S132 S133 S134 S135 S136 S137 S138 L20 L21 S139 S140 S141 S142 S143 S144 S145 S146 S147 S148 S149 S150 S151 S152 S153 S154 S155 S156 S157 S158 S159 S160 S161 S162 S163 S164 S165 S166 S167 S168 S169 S170 S171 L22 L23 S172 S173 S174 S175 S176 S177 S178 L24 L25 S179 S180 S181 L26 L27 S182 S183 S184 S185 L28 L29 S186 S187 S188 S189 S190 S191 S192 S193 S194 S195 S196 S197 S198 S199 S200 S201 S202 S203 S204 S205 S206 S207 S208 S209 S210 S211 S212 S213 L30 L31 S214 S215 S216 S217 S218 S219 S220 S221 S222 S223 S224 S225 S226 S227 S228 S229 S230 S231 S232 L32 L33 S233 S234 S235 S236 S237 S238 S239 S240 S241 S242 S243 S244 S245 S246 S247 S248 S249 S250 S251 S252 S253 S254 S255 | S258 S259 S260 S261 S262 S263 S264 S265 S266 S267 S268 S269 S270 S271 L36 L37 S272 S273 S274 S275 S276 S277 S278 S279 S280 S281 S282 S283 S284 S285 L38 L39 | S286 S287 S288 S289 S290 S291 L40 L41 S292 S293 S294 S295 S296 S297 S298 S299 L42 L43 S300 S301 S302 S303 S304 | S305 S306 S307 S308 L44 L45 S309 L46 L47 S310 S311 S312 S313 S314 S315 S316 S317 S318 S319 | S320 S321 S322 S323 S324 S325 S326 | S327 S328 S329 S330 S331 | S332 S333 S334 S335 S336 S337 S338 S339 S340 S341 S342 S343 S344 S345 S346 S347 S348 | S349 S350 S351 S352 S353 S354 S355 S356 S357 S358 S359 S360 S361 L48 L49 | S377 S378 S379 | S380 S381 S382 | S383 S384 S385 S386 S387 S388 S389 S390 S391 S392 S393 S394 S395 S396 S397 S398 S399 S400 S401 S402 S403 S404 S405 S406 S407 S408 S409 S410 S411 S412 S413 S414 S415 S416 S417 S418 S419 S420 S421 S422 S423 | S435 S436 S437 | S441 S442 S443 S444 L52 L53 S445 S446 S447 S448 S449 S450 S451 S452 S453 S454 S455 S456 S457 S458 S459 S460 S461 S462 S463 S464 S465 S466 S467 S468 S469 S470 S471 S472 S473 S474 S475 S476 S477 S478 S479 S480 S481 S482 | S486 S487 S488 | S489 S490 S491 | S492 S493 S494 S495 | S500 S501 S502 | S506 S507 S508 | S509 S510 L54 L55 S511 S512 L56 L57 S513 S514 S515 S516 S517 S518 | S519 S520 S521 S522 L58 L59 S523 | S524 S525 S526 | S527 S528 S529 | S530 S531 S532 L60 L61 S533 S534 S535 S536 S537 S538 S539 S540 S541 S542 S543 S544 S545 | S546 S547 S548 | S549 S550 S551 | S560 S561 S562 | S566 S567 S568 S569 S570 S571 S572 S573 | S574 S575 S576 | S586 S587 S588 | S604 S605 S606 S607 S608 S609 S610 S611 | S612 S613 S614 S615 | S616 S617 S618 S619 S620 S621 S622 S623 S624 | S629 S630 S631 S632 S633 S634 S635 | S636 S637 S638 S639 S640 S641 S642 S643 S644 | S648 S649 S650 S651 S652 | S653 S654 S655 S656 | S657 S658 S659 S660 S661 S662 S663 S664 S665 S666 S667 S668 S669 S670 S671 S672 S673 S674 | S675 S676 S677 | S678 S679 S680 S681 | S682 S683 S684 S685 | S686 S687 S688 S689 S690 S691 S692 S693 S694 S695 | S696 S697 S698 S699 | S700 S701 S702 S703 | S708 S709 S710 S711 S712 S713 S714 S715 S716 S717 | S718 S719 S720 S721 | S722 S723 S724 | S725 S726 S727 | S731 S732 S733 S734 | S739 S740 S741 S742 | S746 S747 S748 S749 | S750 S751 S752 S753 S754 S755 S756 S757 S758 S759 S760 S761 S762 S763 S764 S765 S766 S767 S768 S769 S770 S771 S772 S773 S774 L62 L63 | S775 S776 S777 | S778 S779 S780 | S781 S782 S783 S784 | S785 S786 S787 | S788 S789 S790 S791 | S792 S793 S794 S795 S796 S797 S798 S799 S800 S801 S802 S803 S804 S805 S806 S807 S808 S809 S810 S811 S812 S813 S814 S815 S816 S817 S818 S819 | S820 S821 S822 S823 | S840 S841 S842 S843 | S844 S845 S846 | S847 S848 S849 | S854 S855 S856 S857 S858 S859 | S860 S861 S862 | S867 S868 S869 | S870 S871 S872 S873 | S874 S875 S876 S877 | S878 S879 S880 S881 | S882 S883 S884 S885 | S923 S924 S925 S926 S927 S928 S929 S930 S931 S932 S933 S934 S935 S936 S937 S938 S939 S940 S941 S942 S943 S944 S945 S946 S947 S948 S949 S950 S951 S952 S953 S954 S955 S956 S957 L64 L65 S958 S959 S960 S961 S962 S963 S964 S965 | S992 S993 S994 L66 L67 S995 S996 S997 S998 S999 S1000 S1001 S1002 S1003 S1004 S1005 S1006 S1007 L68 L69 S1008 S1009 S1010 S1011 S1012 S1013 S1014 S1015 S1016 S1017 S1018 S1019 S1020 S1021 S1022 S1023 | S1349 S1350 S1351 | S1463 S1464 S1465 S1466 S1467 S1468 S1469 | S1483 S1484 S1485 S1486 S1487 | S1773 S1774 S1775 S1776 | S1787 S1788 S1789 S1790
sketch "Sketch4" plane through (0, 0, 0) normal (0, 0, 1) x (1, 0, 0)
